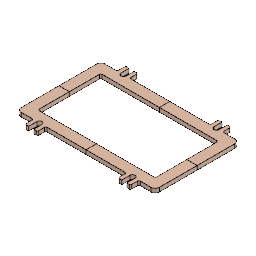
Task1b v0 (Autodesk Fusion 360 design; units mm, degrees)
Autodesk Fusion 360 part; units mm, degrees
sketch "Sketch1" plane through (0, 0, 0) normal (0, 1, 0) x (1, 0, 0)
  line L0 (0, 0) -> (0, -100)
  line L1 (0, -100) -> (39, -100)
  line L2 (39, -100) -> (39, -120)
  line L3 (39, -120) -> (48, -120)
  line L4 (48, -120) -> (48, -100)
  line L5 (48, -100) -> (60, -100)
  line L6 (60, -100) -> (60, -120)
  line L7 (60, -120) -> (69, -120)
  line L8 (69, -120) -> (69, -100)
  line L9 (69, -100) -> (165, -100)
  line L10 (165, -100) -> (165, -75)
  line L11 (165, -75) -> (25, -75)
  line L12 (25, -75) -> (25, 0)
  line L13 (25, 0) -> (0, 0)
  line L14 (165, -75) -> (165, 0) construction
  line L15 (165, 0) -> (25, 0) construction
  dimension "d9" = 100
  dimension "d10" = 39
  dimension "d11" = 20
  dimension "d12" = 9
  dimension "d13" = 12
  dimension "d14" = 9
  dimension "d15" = 96
  dimension "d16" = 25
  dimension "d17" = 140
  dimension "d18" = 75
  constraint coincident L0.start L13.end
  constraint vertical L0
  constraint perpendicular L0 L1
  constraint perpendicular L1 L2
  constraint perpendicular L0 L3
  constraint perpendicular L3 L4
  constraint perpendicular L4 L5
  constraint perpendicular L5 L6
  constraint perpendicular L6 L7
  constraint perpendicular L7 L8
  constraint perpendicular L0 L9
  constraint perpendicular L9 L10
  constraint perpendicular L10 L11
  constraint perpendicular L9 L12
  constraint perpendicular L0 L13
  constraint perpendicular L11 L14
  constraint perpendicular L14 L15
  measures "d9" distance of L0.start L0.end
  measures "d10" distance of L0.end L1.end
  measures "d11" distance of L1.end L2.end
  measures "d12" distance of L2.end L3.end
  measures "d13" distance of L4.end L5.end
  measures "d14" distance of L6.end L7.end
  measures "d15" distance of L8.end L9.end
  measures "d16" distance of L9.end L10.end
  measures "d17" distance of L10.end L11.end
  measures "d18" distance of L11.end L12.end
sketch "Sketch2" plane through (0, 0, 0) normal (0, 1, 0) x (1, 0, 0)
sketch "Sketch3" plane through (82.5, 0, 60) normal (0, 1, 0) x (1, 0, 0)
extrude "Extrude1" add sketch "Sketch1" along normal blind 10 makes body 1
fillet "Fillet1" radius 10 1 edges at (0, 5, 100) on bodies 1
fillet "Fillet2" radius 3 1 edges at (25, 5, 75) on bodies 1
fillet "Fillet3" radius 3 4 edges at (69, 5, 100) (39, 5, 100) (39, 5, 120) (69, 5, 120) on bodies 1
sketch "Sketch4" plane through (0, 10, 0) normal (0, 1, 0) x (-1, 0, 0)
  arc A0 (-66, 120) -> (-69, 117) centre (-66, 117) ccw
  line L0 (-69, 117) -> (-69, 103)
  arc A1 (-72, 100) -> (-69, 103) centre (-72, 103) ccw
  line L1 (-72, 100) -> (-165, 100)
  line L2 (-165, 100) -> (-165, 75)
  line L3 (-165, 75) -> (-28, 75)
  arc A2 (-25, 72) -> (-28, 75) centre (-28, 72) ccw
  line L4 (-25, 72) -> (-25, 0)
  line L5 (-25, 0) -> (0, 0)
  line L6 (0, 0) -> (0, 90)
  arc A3 (0, 90) -> (-10, 100) centre (-10, 90) ccw
  line L7 (-10, 100) -> (-36, 100)
  arc A4 (-39, 103) -> (-36, 100) centre (-36, 103) ccw
  line L8 (-39, 103) -> (-39, 117)
  arc A5 (-39, 117) -> (-42, 120) centre (-42, 117) ccw
  line L9 (-42, 120) -> (-48, 120)
  line L10 (-48, 120) -> (-48, 100)
  line L11 (-48, 100) -> (-60, 100)
  line L12 (-60, 100) -> (-60, 120)
  line L13 (-60, 120) -> (-66, 120)
  circle A6 centre (-54, 100) radius 6
  constraint midpoint L11 A6.centre
  constraint coincident L11.end A6
extrude "Extrude2" cut sketch "Sketch4" against normal blind 20 contours L11 A6 picked at (-54.445, 98.0501) bodies 1
mirror "Mirror1" about plane through (0, 0, 0) normal (0, 0, 1) of bodies 1 makes body 2
move_face "MoveFace1" by (165, 0, 0) 2 faces at (8.3333, 10, 54) (8.3333, 10, -54) on bodies 1 2
move_body "Move1" bodies 1 2 to x (1, 0, 0) y (0, 1, 0) z (0, 0, 1) at (-165, 0, 0)
mirror "Mirror2" about plane through (0, 0, 0) normal (1, 0, 0) of bodies 1 2 makes body 3 at (156.6667, 0, -54) makes body 4 at (156.6667, 0, 54)
